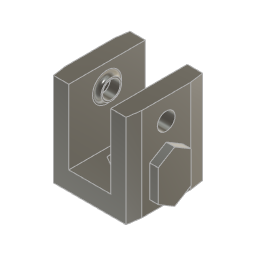
20t pulley cr6 front (Autodesk Fusion 360 design; units mm, degrees)
Autodesk Fusion 360 part; units mm, degrees
sketch "Sketch1" plane through (0, 0, 0) normal (0, 0, 1) x (1, 0, 0)
  line L0 (9.75, -9.75) -> (-9.75, -9.75)
  line L1 (-9.75, -9.75) -> (-9.75, 9.75)
  line L2 (-9.75, 9.75) -> (9.75, 9.75)
  line L3 (9.75, 9.75) -> (9.75, -9.75)
  line L4 (9.75, -9.75) -> (-9.75, 9.75) construction
  line L5 (-9.75, -9.75) -> (9.75, 9.75) construction
  line L6 (0, 9.75) -> (0, -9.75) construction
  dimension "d1" = 19.5
  dimension "d2" = 19.5
  constraint horizontal L0
  constraint perpendicular L0 L1
  constraint parallel L0 L2
  constraint parallel L1 L3
  constraint coincident L4 origin
  constraint coincident L5 origin
  constraint midpoint L2 L6.start
  constraint midpoint L0 L6.end
  measures "d1" distance of L1.end L2.end
  measures "d2" distance of L0.end L1.end
extrude "Extrude1" add sketch "Sketch1" along normal blind 4.81
sketch "Sketch3" plane through (0, 0, 0) normal (0, 0, -1) x (1, 0, 0)
  line L0 (-9.75, -9.75) -> (9.75, -9.75)
  line L1 (9.75, -9.75) -> (9.75, 9.75)
  line L2 (9.75, 9.75) -> (-9.75, 9.75)
  line L3 (-9.75, 9.75) -> (-9.75, -9.75)
  circle A0 centre (0, 0) radius 5.975
  circle A1 centre (0, 0) radius 2.5
  dimension "d5" = 11.95
  dimension "d6" = 5
  constraint coincident A0.centre A1.centre
  constraint concentric A0 A1
  measures "d5" diameter of A0
  measures "d6" diameter of A1
extrude "Extrude2" cut sketch "Sketch3" against normal through all contours A1
extrude "Extrude3" add sketch "Sketch3" along normal blind 1.05 contours A0 | A1
sketch "Sketch4" plane through (0, 0, 4.81) normal (0, 0, 1) x (-1, 0, 0)
  circle A0 centre (0, 0) radius 2.5
  line L0 (-9.75, -9.75) -> (9.75, -9.75)
  line L1 (9.75, -9.75) -> (9.75, 9.75)
  line L2 (9.75, 9.75) -> (-9.75, 9.75)
  line L3 (-9.75, 9.75) -> (-9.75, -9.75)
  line L4 (0, -9.75) -> (0, 9.75) construction
  line L5 (-9.75, -9.75) -> (-5.35, -9.75)
  line L6 (-5.35, -9.75) -> (-5.35, 9.75)
  line L7 (-5.35, 9.75) -> (-9.75, 9.75)
  line L8 (-9.75, 9.75) -> (-9.75, -9.75)
  line L9 (5.35, -9.75) -> (5.35, 9.75)
  line L10 (9.75, -9.75) -> (5.35, -9.75)
  line L11 (9.75, 9.75) -> (9.75, -9.75)
  line L12 (5.35, 9.75) -> (9.75, 9.75)
  dimension "d37" = 3.5
  dimension "d38" = 0.5
  dimension "d39" = 0.5
  dimension "d40" = 3.5
  constraint midpoint L0 L4.start
  constraint midpoint L2 L4.end
  constraint horizontal L5
  constraint vertical L6
  constraint horizontal L7
  constraint vertical L8
  constraint coincident L0.start L3.end
  constraint symmetric L4 L0.start L0.end
  constraint symmetric L4 L5.end L9.start
  constraint symmetric L4 L6.end L9.end
  constraint symmetric L4 L2.end L1.end
  measures "d10" distance of L0.start L5.end
extrude "Extrude4" add sketch "Sketch4" along normal blind 18.9 contours L0 L2 L3 L5 L6 L7 L8 | L0 L1 L2 L9 L10 L11 L12
ref_plane "WorkPlane1" through (0, 0, 11.855) normal (-1, 0, 0) x (0, -1, 0)
sketch "Sketch5" plane through (9.75, 0, 0) normal (1, 0, 0) x (0, 1, 0)
  line L0 (-9.75, 0) -> (9.75, 0)
  line L1 (9.75, 0) -> (9.75, 23.71)
  line L2 (9.75, 23.71) -> (-9.75, 23.71)
  line L3 (-9.75, 23.71) -> (-9.75, 0)
  circle A0 centre (0, 18.25) radius 2.5
  dimension "d13" = 5
  dimension "d14" = 18.25
  measures "d13" diameter of A0
  measures "d14" distance of origin A0.centre
sketch "Sketch6" plane through (-9.75, 0, 0) normal (-1, 0, 0) x (0, -1, 0)
  line L0 (-9.75, 0) -> (9.75, 0)
  line L1 (9.75, 0) -> (9.75, 23.71)
  line L2 (9.75, 23.71) -> (-9.75, 23.71)
  line L3 (-9.75, 23.71) -> (-9.75, 0)
  circle A0 centre (0, 18.25) radius 2.5
sketch "Sketch7" plane through (-5.35, 0, 0) normal (1, 0, 0) x (0, 1, 0)
  line L0 (-9.75, 4.81) -> (9.75, 4.81)
  line L1 (9.75, 4.81) -> (9.75, 23.71)
  line L2 (9.75, 23.71) -> (-9.75, 23.71)
  line L3 (-9.75, 23.71) -> (-9.75, 4.81)
  circle A0 centre (0, 18.25) radius 2.5
  circle A1 centre (0, 18.25) radius 2.6
  dimension "d15" = 5.2
  constraint concentric A0 A1
  measures "d15" diameter of A1
extrude "Extrude5" add sketch "Sketch7" along normal blind 1.1 contours A0 | A1
fillet "Fillet1" radius 1.1 1 edges at (-5.35, -2.4241, 19.1902)
mirror "Mirror1" about plane through (0, 0, 11.855) normal (-1, 0, 0) of 2 faces at (-5.3488, -2.1292, 21.2115) (-4.25, -1.2564, 18.8127)
hole "Hole1" at (9.75, 0, 18.25) direction (-1, 0, 0) diameter 4.5 end through all
extrude "Extrude6" [suppressed]
sketch "Sketch9" plane through (9.75, 0, 0) normal (1, 0, 0) x (0, 1, 0)
  circle A0 centre (0, 18.25) radius 2.25
  line L0 (-9.75, 0) -> (9.75, 0)
  line L1 (9.75, 0) -> (9.75, 23.71)
  line L2 (9.75, 23.71) -> (-9.75, 23.71)
  line L3 (-9.75, 23.71) -> (-9.75, 0)
  line L4 (0, 0) -> (0, 23.71) construction
  line L5 (-4.2, 0.5) -> (4.2, 0.5)
  line L6 (4.2, 0.5) -> (4.2, 13.62)
  line L7 (4.2, 13.62) -> (-4.2, 13.62)
  line L8 (-4.2, 13.62) -> (-4.2, 0.5)
  line L9 (-4.2, 0.5) -> (4.2, 13.62) construction
  line L10 (4.2, 0.5) -> (-4.2, 13.62) construction
  line L11 (0, 0.5) -> (4.2, 3)
  line L12 (4.2, 7.06) -> (-4.2, 7.06) construction
  line L13 (0, 13.62) -> (4.2, 11.12)
  line L14 (0, 13.62) -> (-4.2, 11.12)
  line L15 (0, 0.5) -> (-4.2, 3)
  point P0 (0, 7.06)
  dimension "d27" = 8.4
  dimension "d28" = 13.12
  dimension "d29" = 2.5
  dimension "d32" = 0.5
  constraint coincident L4.start origin
  constraint midpoint L2 L4.end
  constraint horizontal L5
  constraint perpendicular L5 L6
  constraint parallel L5 L7
  constraint parallel L6 L8
  constraint coincident L9 P0
  constraint coincident L10 P0
  constraint coincident L4 P0
  constraint midpoint L5 L11.start
  constraint coincident L6 L11.end
  constraint midpoint L6 L12.start
  constraint midpoint L8 L12.end
  constraint symmetric L11.start L12 L13.start
  constraint symmetric L11.end L12 L13.end
  constraint symmetric L4 L11.start L15.start
  constraint symmetric L4 L11.end L15.end
  constraint symmetric L4 L13.start L14.start
  constraint symmetric L4 L13.end L14.end
  measures "d27" distance of L6.end L7.end
  measures "d28" distance of L5.end L6.end
  measures "d29" distance of L5.end L11.end
  measures "d32" distance of L0 L5
extrude "Extrude7" add sketch "Sketch9" along normal blind 2.15 contours L6 L8 L11 L13 L14 L15
mirror "Mirror2" about plane through (0, 0, 11.855) normal (-1, 0, 0) of "Extrude7"
chamfer "Chamfer2" distance 3.5 distance2 0.5 2 edges at (-9.75, -9.75, 11.855) (9.75, 9.75, 11.855) measured on face at (-9.75, -7.9, 11.61) measured on face at (9.75, 7.9, 11.61)
chamfer "Chamfer2" distance 0.5 distance2 3.5 2 edges at (-9.75, 9.75, 11.855) (9.75, -9.75, 11.855) measured on face at (-1.7833, 9.75, 1.6033) measured on face at (1.7833, -9.75, 1.6033)
sketch "Sketch11" plane through (0, 0, 4.81) normal (0, 0, 1) x (-1, 0, 0)
  circle A0 centre (0, 0) radius 2.5
  line L0 (5.35, -9.75) -> (5.35, 9.75)
  line L1 (5.35, 9.75) -> (-5.35, 9.75)
  line L2 (-5.35, 9.75) -> (-5.35, -9.75)
  line L3 (-5.35, -9.75) -> (5.35, -9.75)
  line L4 (-3.4, -1.963) -> (0, -3.926)
  line L5 (0, -3.926) -> (3.4, -1.963)
  line L6 (3.4, -1.963) -> (3.4, 1.963)
  line L7 (3.4, 1.963) -> (0, 3.926)
  line L8 (0, 3.926) -> (-3.4, 1.963)
  line L9 (-3.4, 1.963) -> (-3.4, -1.963)
  dimension "d44" = 3.4
  constraint coincident A0.centre origin
  measures "d44" distance of A0.centre L9
extrude "Extrude9" cut sketch "Sketch11" against normal blind 3 contours L4 L5 L6 L7 L8 L9
hole "Hole2" at (0, 0, -1.05) direction (0, 0, 1) diameter 4.5 depth 5.5 tip angle 118
sketch "Sketch12" plane through (-9.75, 0, 0) normal (-1, 0, 0) x (0, -1, 0)
  line L0 (0, 0.5) -> (-4.2, 3)
  line L1 (-4.2, 3) -> (-4.2, 11.12)
  line L2 (-4.2, 11.12) -> (0, 13.62)
  line L3 (0, 13.62) -> (4.2, 11.12)
  line L4 (4.2, 11.12) -> (4.2, 3)
  line L5 (4.2, 3) -> (0, 0.5)
  circle A0 centre (0, 18.25) radius 2.25
  line L6 (-6.25, 23.71) -> (-6.25, 0)
  line L7 (-6.25, 0) -> (6.25, 0)
  line L8 (6.25, 0) -> (6.25, 23.71)
  line L9 (6.25, 23.71) -> (-6.25, 23.71)
  line L10 (1.963, 14.85) -> (3.926, 18.25)
  line L11 (3.926, 18.25) -> (1.963, 21.65)
  line L12 (1.963, 21.65) -> (-1.963, 21.65)
  line L13 (-1.963, 21.65) -> (-3.926, 18.25)
  line L14 (-3.926, 18.25) -> (-1.963, 14.85)
  line L15 (-1.963, 14.85) -> (1.963, 14.85)
  point P0 (0, 18.25)
  dimension "d50" = 3.4
  constraint coincident P0 A0.centre
  measures "d50" distance of P0 L15
extrude "Extrude10" cut sketch "Sketch12" against normal blind 3 contours L10 L11 L12 L13 L14 L15
